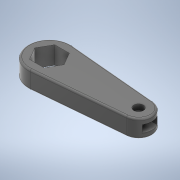
# Autodesk Inventor part: Crank
Saved by Autodesk Inventor 2020.2 (Build 242310000, 310)
## iProperties
Created: 2021-06-25
Part Number: Crank
Material: Generic
Document SubType Name: Modeling
Designer: JK
Density: 1 g/cm^3
Appearance: Smooth - Black
Author: JK
Autodesk Inventor part; units mm, degrees
ref_plane "XZ Plane" through (0, 0, 0) normal (0, 1, 0) x (-1, 0, 0)
ref_plane "XY Plane" through (0, 0, 0) normal (0, 0, 1) x (1, 0, 0)
sketch "Sketch1" plane through (0, 0, 0) normal (0, 1, 0) x (-1, 0, 0)
  circle A0 centre (0, 0) radius 4
  circle A1 centre (0, 0) radius 12
  dimension "d0" = 8
  dimension "d1" = 24
  constraints: 2 centre point, 2 coincident
  measures "d0" diameter of A0
  measures "d1" diameter of A1
extrude "Extrusion1" add sketch "Sketch1" along normal blind 10
sketch "Sketch2" plane through (0, 10, 0) normal (0, 1, 0) x (1, 0, 0)
  circle A0 centre (0, 0) radius 12 projected
  line L0 (1.08, 11.9513) -> (50.675, 7.4696)
  circle A1 centre (50, 0) radius 7.5
  line L1 (50.675, -7.4696) -> (1.08, -11.9513)
  circle A2 centre (50, 0) radius 2.7
  circle A3 centre (0, 0) radius 12 projected
  point P0 (3.9985, -10.2475)
  point P1 (1.1339, 10.9414)
  dimension "d4" = 50
  dimension "d5" = 15
  dimension "d6" = 5.4
  constraints: 4 end point, 4 point on circle, 4 tangent, 2 centre point, 1 coincident, 1 horizontal alignment
  measures "d4" distance of A1.centre point (0, 0)
  measures "d5" diameter of A1
  measures "d6" diameter of A2
extrude "Extrusion2" add sketch "Sketch2" against normal up to surface (10 mm away) contours A0 L0 A1 L1 | A1
sketch "Sketch3" plane through (0, 10, 0) normal (0, 1, 0) x (1, 0, 0)
  circle A0 centre (0, 0) radius 7.1
  line L0 (8.1984, 0) -> (4.0992, -7.1)
  line L1 (4.0992, -7.1) -> (-4.0992, -7.1)
  line L2 (-4.0992, -7.1) -> (-8.1984, 0)
  line L3 (-8.1984, 0) -> (-4.0992, 7.1)
  line L4 (-4.0992, 7.1) -> (4.0992, 7.1)
  line L5 (4.0992, 7.1) -> (8.1984, 0)
  dimension "d9" = 14.2
  constraints: 12 end point, 2 coincident, 1 centre point, 1 tangent, 13 other
  measures "d9" diameter of A0
extrude "Extrusion3" cut sketch "Sketch3" against normal blind 10
ref_plane "Work Plane1" through (57.5, 10, 0) normal (1, 0, 0) x (0, 1, 0)
sketch "Sketch4" plane through (57.5, 10, 0) normal (1, 0, 0) x (0, 1, 0)
  line L0 (-2.9, -4.1) -> (-7.1, -4.1)
  line L1 (-7.1, -4.1) -> (-7.1, 4.1)
  line L2 (-7.1, 4.1) -> (-2.9, 4.1)
  line L3 (-2.9, 4.1) -> (-2.9, -4.1)
  line L4 (0, 0) -> (-10, 0) projected
  line L5 (-2.9, -4.1) -> (-7.1, 4.1) construction
  line L6 (-7.1, -4.1) -> (-2.9, 4.1) construction
  point P0 (-5, 0)
  dimension "d12" = 4.2
  dimension "d13" = 8.2
  constraints: 12 end point, 3 midpoint, 2 parallel, 1 horizontal, 1 perpendicular
  measures "d12" distance between parallel lines of L1 L3
  measures "d13" distance between parallel lines of L2 L0
extrude "Extrusion4" cut sketch "Sketch4" against normal blind 12.5
chamfer "Chamfer1" distance 3 angle 30 2 edges at (45, 5, -4.1) (45, 5, 4.1) measured on face at (45, 4.3, -1.3667)
fillet "Fillet1" radius 1 8 edges at (-12, 0, 0) (25.8775, 0, -9.7104) (57.5, 0, 0) (25.8775, 0, 9.7104) (57.5, 10, 0) (25.8775, 10, -9.7104) (-12, 10, 0) (25.8775, 10, 9.7104)
body "Solid1"
